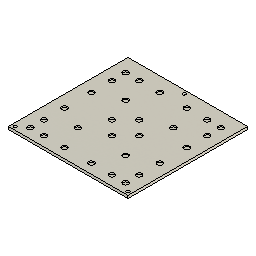
V2, Build plate with pockets for magnets (Autodesk Fusion 360 design; units mm, degrees)
Autodesk Fusion 360 part; units mm, degrees
sketch "Sketch1" plane through (0, 0, 0) normal (0, 0, 1) x (1, 0, 0)
  line L0 (165, 165) -> (-165, 165) construction
  line L1 (-165, 165) -> (-165, -165) construction
  line L2 (-165, -165) -> (165, -165) construction
  line L3 (165, -165) -> (165, 165) construction
  line L4 (165, 165) -> (-165, -165) construction
  line L5 (-165, 165) -> (165, -165) construction
  line L6 (-175, 175) -> (-175, -175)
  line L7 (-175, -175) -> (175, -175)
  line L8 (175, -175) -> (175, 175)
  line L9 (175, 175) -> (-175, 175)
  dimension "d636" = 330
  dimension "d637" = 330
  dimension "d638" = 10
  constraint horizontal L0
  constraint perpendicular L0 L1
  constraint parallel L0 L2
  constraint parallel L1 L3
  constraint coincident L4 origin
  constraint coincident L5 origin
  measures "d636" distance of L0.end L1.end
  measures "d637" distance of L1.end L2.end
extrude "Extrude1" add sketch "Sketch1" along normal blind 8 makes body 1
sketch "Sketch2" plane through (0, 0, 8) normal (0, 0, 1) x (-1, 0, 0)
  line L0 (-175, -175) -> (175, -175)
  line L1 (175, -175) -> (175, 175)
  line L2 (175, 175) -> (-175, 175)
  line L3 (-175, 175) -> (-175, -175)
  line L4 (-165, 165) -> (165, 165) construction
  line L5 (165, 165) -> (165, -165) construction
  line L6 (165, -165) -> (-165, -165) construction
  line L7 (-165, -165) -> (-165, 165) construction
  line L8 (-165, 165) -> (165, -165) construction
  line L9 (165, 165) -> (-165, -165) construction
  point P0 (0, -165)
  dimension "d641" = 330
  dimension "d642" = 330
  constraint horizontal L4
  constraint perpendicular L4 L5
  constraint parallel L4 L6
  constraint parallel L5 L7
  constraint coincident L8 origin
  constraint coincident L9 origin
  constraint midpoint L6 P0
  measures "d641" distance of L4.end L5.end
  measures "d642" distance of L5.end L6.end
hole "Hole1" at (0, 165, 8) at (165, -165, 8) at (-165, -165, 8) direction (0, 0, -1) diameter 3.332 end through all countersink diameter 9.4 countersink angle 90 bodies 1
thread "Thread1" "ISO Metric profile 4.0 M4x0.7 M4x0.7 6H" major diameter 4.1095 minor diameter 3.332 pitch 0.7 angle 60 resizes the face on face at (-1.6037, 164.5488, 3.3107) on face at (-166.0709, -166.2762, 3.3107) on face at (163.9291, -166.2762, 3.3107) on bodies 1
sketch "Sketch3" plane through (0, 0, 8) normal (0, 0, 1) x (-1, 0, 0)
  circle A0 centre (-165, 165) radius 4.7
  circle A1 centre (0, -165) radius 4.7
  circle A2 centre (165, 165) radius 4.7
  line L0 (-175, -175) -> (175, -175)
  line L1 (175, -175) -> (175, 175)
  line L2 (175, 175) -> (-175, 175)
  line L3 (-175, 175) -> (-175, -175)
  line L4 (139.5, -132.5) -> (-139.5, -132.5) construction
  line L5 (-139.5, -132.5) -> (-139.5, 146.5) construction
  line L6 (-139.5, 146.5) -> (139.5, 146.5) construction
  line L7 (139.5, 146.5) -> (139.5, -132.5) construction
  circle A3 centre (139.5, 106.5) radius 7.9
  circle A4 centre (99.5, 146.5) radius 7.9
  line L8 (155, -148) -> (-155, -148) construction
  line L9 (-155, -148) -> (-155, 162) construction
  line L10 (-155, 162) -> (155, 162) construction
  line L11 (155, 162) -> (155, -148) construction
  line L12 (155, -148) -> (-155, 162) construction
  line L13 (-139.5, -132.5) -> (139.5, 146.5) construction
  line L14 (0, 0) -> (0, 7) construction
  circle A5 centre (139.5, 146.5) radius 7.9
  circle A6 centre (39.5, 146.5) radius 7.9
  circle A7 centre (139.5, 46.5) radius 7.9
  circle A8 centre (70, 77) radius 7.9
  circle A9 centre (40, 7) radius 7.9
  line L15 (139.5, 7) -> (-139.5, 7) construction
  circle A10 centre (0, 7) radius 5 construction
  point P0 (0, 7)
  dimension "d6" = 15.8
  dimension "d9" = 310
  dimension "d10" = 7
  dimension "d13" = 15.5
  dimension "d14" = 40
  dimension "d15" = 40
  dimension "d23" = 60
  dimension "d24" = 60
  dimension "d25" = 30
  dimension "d26" = 40
  dimension "d29" = 10
  constraint horizontal L4
  constraint vertical L5
  constraint horizontal L6
  constraint vertical L7
  constraint coincident L7 A3.centre
  constraint coincident L6 A4.centre
  constraint horizontal L8
  constraint vertical L9
  constraint horizontal L10
  constraint vertical L11
  constraint midpoint L12 L13
  constraint coincident L14.start origin
  constraint midpoint L12 P0
  constraint vertical L14
  constraint equal L8 L11
  constraint equal L6 L7
  constraint coincident L6.end L7.start
  constraint equal A3 A5
  constraint equal A3 A4
  constraint coincident L6 A6.centre
  constraint equal A3 A6
  constraint coincident L7 A7.centre
  constraint equal A3 A7
  constraint coincident L13 A8.centre
  constraint equal A3 A8
  constraint midpoint L7 L15.start
  constraint midpoint L5 L15.end
  constraint coincident A9.centre L15
  constraint equal A3 A9
  constraint coincident P0 L14.end
  measures "d6" diameter of A3
  measures "d9" distance of L8.start L8.end
  measures "d10" distance of L14.start P0
  measures "d13" distance of L7 L11
  measures "d14" distance of L6.end A4.centre
  measures "d15" distance of L6.end A3.centre
  measures "d23" distance of A4.centre A6.centre
  measures "d24" distance of A3.centre A7.centre
  measures "d25" horizontal distance of A8.centre A9.centre
  measures "d26" horizontal distance of A9.centre L14.start
  measures "d29" diameter of A10
extrude "Extrude2" cut sketch "Sketch3" against normal blind 3.4 contours A3 | A4 | A5 | A6 | A7 | A8 | A9 bodies 1
pattern_circular "C-Pattern1" count 4 over 360 about axis through (0, -7, 8) along (0, 0, 1) of "Extrude2"
sketch "Sketch1 (2)" plane through (0, 0, 0) normal (0, 0, 1) x (1, 0, 0) in component "magnet"
  circle A0 centre (0, 0) radius 7.5
  dimension "d41" = 15
  constraint coincident A0.centre origin
  measures "d41" diameter of A0
extrude "Extrude1'" add sketch "Sketch1 (2)" along normal blind 3 separate body makes body 2 in component "magnet"
component_pattern "component pattern"
component "magnet" placed x (1, 0, 0) y (0, 1, 0) z (0, 0, 1) at (-139.5, -146.5, 5)
component "magnet" placed x (1, 0, 0) y (0, 1, 0) z (0, 0, 1) at (-139.5, -106.5, 5)
component "magnet" placed x (1, 0, 0) y (0, 1, 0) z (0, 0, 1) at (-139.5, -46.5, 5)
component "magnet" placed x (1, 0, 0) y (0, 1, 0) z (0, 0, 1) at (-70, -77, 5)
component "magnet" placed x (1, 0, 0) y (0, 1, 0) z (0, 0, 1) at (-99.5, -146.5, 5)
component "magnet" placed x (1, 0, 0) y (0, 1, 0) z (0, 0, 1) at (-39.5, -146.5, 5)
component "magnet" placed x (1, 0, 0) y (0, 1, 0) z (0, 0, 1) at (-40, -7, 5)
component "magnet" placed x (0, 1, 0) y (-1, 0, 0) z (0, 0, 1) at (139.5, -146.5, 5)
component "magnet" placed x (0, 1, 0) y (-1, 0, 0) z (0, 0, 1) at (99.5, -146.5, 5)
component "magnet" placed x (0, 1, 0) y (-1, 0, 0) z (0, 0, 1) at (39.5, -146.5, 5)
component "magnet" placed x (0, 1, 0) y (-1, 0, 0) z (0, 0, 1) at (70, -77, 5)
component "magnet" placed x (0, 1, 0) y (-1, 0, 0) z (0, 0, 1) at (139.5, -106.5, 5)
component "magnet" placed x (0, 1, 0) y (-1, 0, 0) z (0, 0, 1) at (139.5, -46.5, 5)
component "magnet" placed x (0, 1, 0) y (-1, 0, 0) z (0, 0, 1) at (0, -47, 5)
component "magnet" placed x (-1, 0, 0) y (0, -1, 0) z (0, 0, 1) at (139.5, 132.5, 5)
component "magnet" placed x (-1, 0, 0) y (0, -1, 0) z (0, 0, 1) at (139.5, 92.5, 5)
component "magnet" placed x (-1, 0, 0) y (0, -1, 0) z (0, 0, 1) at (139.5, 32.5, 5)
component "magnet" placed x (-1, 0, 0) y (0, -1, 0) z (0, 0, 1) at (70, 63, 5)
component "magnet" placed x (-1, 0, 0) y (0, -1, 0) z (0, 0, 1) at (99.5, 132.5, 5)
component "magnet" placed x (-1, 0, 0) y (0, -1, 0) z (0, 0, 1) at (39.5, 132.5, 5)
component "magnet" placed x (-1, 0, 0) y (0, -1, 0) z (0, 0, 1) at (40, -7, 5)
component "magnet" placed x (0, -1, 0) y (1, 0, 0) z (0, 0, 1) at (-139.5, 132.5, 5)
component "magnet" placed x (0, -1, 0) y (1, 0, 0) z (0, 0, 1) at (-99.5, 132.5, 5)
component "magnet" placed x (0, -1, 0) y (1, 0, 0) z (0, 0, 1) at (-39.5, 132.5, 5)
component "magnet" placed x (0, -1, 0) y (1, 0, 0) z (0, 0, 1) at (-70, 63, 5)
component "magnet" placed x (0, -1, 0) y (1, 0, 0) z (0, 0, 1) at (-139.5, 92.5, 5)
component "magnet" placed x (0, -1, 0) y (1, 0, 0) z (0, 0, 1) at (-139.5, 32.5, 5)
component "magnet" placed x (0, -1, 0) y (1, 0, 0) z (0, 0, 1) at (0, 33, 5)
equation "d636 = y_balljoint_distance"
equation "d637 = x_balljoint_distance"
equation "d641 = y_balljoint_distance"
equation "d642 = x_balljoint_distance"
equation "x_balljoint_distance = 330 mm"
equation "y_balljoint_distance = x_balljoint_distance"
equation "MagnetDia = 15 mm"
equation "d6 = PocketDia"
equation "PrintSurface = 310 mm"
equation "d9 = PrintSurface"
equation "MagnetThickness = 3 mm"
equation "MagnetOffset = MagnetDia / 2 + 8 mm"
equation "d13 = MagnetOffset"
equation "d27 = -PocketDepth"
equation "d41 = MagnetDia"
equation "d42 = MagnetThickness"
equation "GlueSpace = 0.4 mm"
equation "PocketDia = MagnetDia + GlueSpace * 2"
equation "PocketDepth = MagnetThickness + GlueSpace"
named bodies: "Buildplate 350x350x8_1x"
